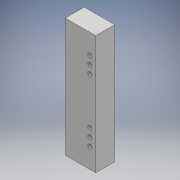
# Autodesk Inventor part: RodBase
Saved by Autodesk Inventor 2017 SP1 (Build 210196100, 196)
## iProperties
Created: 2017-10-17
Part Number: RodBase
Material: Generic
Document SubType Name: Modeling
Designer: 1452927
Density: 1 g/cm^3
Appearance: Default
Author: 1452927
Autodesk Inventor part; units mm, degrees
ref_plane "YZ Plane" through (0, 0, 0) normal (1, 0, 0) x (0, 1, 0)
ref_plane "XZ Plane" through (0, 0, 0) normal (0, 1, 0) x (-1, 0, 0)
ref_plane "XY Plane" through (0, 0, 0) normal (0, 0, 1) x (1, 0, 0)
sketch "Sketch1" plane through (0, 0, 0) normal (0, 1, 0) x (-1, 0, 0)
  line L0 (19.05, -83) -> (19.05, 83)
  line L1 (-19.05, 83) -> (-19.05, -83)
  circle A0 centre (0, 0) radius 11.5094
  line L2 (0, 0) -> (-0.4877, 3.251) construction
  line L3 (0, 0) -> (0, 44.45) construction
  line L4 (0, 0) -> (0, -44.45) construction
  circle A1 centre (0, 44.45) radius 3.5719
  circle A2 centre (0, -44.45) radius 3.5719
  line L5 (19.05, 83) -> (-19.05, 83)
  line L6 (19.05, -83) -> (-19.05, -83)
  dimension "d2" = 23.0188
  dimension "d4" = 44.45
  dimension "d5" = 44.45
  dimension "d6" = 7.1437
  dimension "d7" = 7.1437
  constraints: 14 end point, 3 centre point, 3 coincident, 2 perpendicular, 2 vertical, 1 parallel
  measures "d2" diameter of A0
  measures "d4" distance of L2.start L3.end
  measures "d5" distance of L2.start L4.end
  measures "d6" diameter of A1
  measures "d7" diameter of A2
extrude "Extrusion1" add sketch "Sketch1" along normal blind 25.4
sketch "Sketch6" plane through (0, 0, 0) normal (0, -1, 0) x (1, 0, 0)
  circle A0 centre (0, 44.45) radius 3.5719 projected
  circle A1 centre (0, 44.45) radius 3.5719
  circle A2 centre (0, -44.45) radius 3.5719 projected
  circle A3 centre (0, -44.45) radius 3.5719
  circle A4 centre (0, 0) radius 5.1594
  circle A5 centre (0, 0) radius 11.5094
  dimension "d102" = 35.7188
  constraints: 4 centre point, 4 coincident
sketch "Sketch13" plane through (0, 25.4, 0) normal (0, 1, 0) x (1, 0, 0)
  line L0 (-19.05, -83) -> (19.05, -83) construction
  line L1 (19.05, 83) -> (-19.05, 83) construction
  circle A0 centre (8.0969, -34) radius 1.8
  circle A1 centre (8.0969, -27) radius 1.8
  circle A2 centre (8.0969, -20) radius 1.8
  circle A3 centre (8.0969, 20) radius 1.8
  circle A4 centre (8.0969, 27) radius 1.8
  circle A5 centre (8.0969, 34) radius 1.8
  circle A6 centre (0, 0) radius 11.5094 projected
  line L2 (-19.05, 83) -> (-19.05, -83) projected
  line L3 (-19.05, -83) -> (-13.0969, -83)
  line L4 (-13.0969, -83) -> (-13.0969, 83)
  line L5 (-13.0969, 83) -> (-19.05, 83)
  line L6 (-19.05, 83) -> (-19.05, -83)
  line L7 (19.05, -83) -> (13.0969, -83)
  line L8 (13.0969, -83) -> (13.0969, 83)
  line L9 (13.0969, 83) -> (19.05, 83)
  line L10 (19.05, 83) -> (19.05, -83)
  line L11 (13.0969, -83) -> (3.0969, -83) construction
  line L12 (3.0969, -83) -> (3.0969, 83) construction
  line L13 (3.0969, 83) -> (13.0969, 83) construction
  line L14 (13.0969, 83) -> (13.0969, -83) construction
  line L15 (8.0969, -83) -> (8.0969, 83) construction
  dimension "d82" = 3.6
  dimension "d83" = 3.6
  dimension "d84" = 3.6
  dimension "d85" = 3.6
  dimension "d86" = 3.6
  dimension "d87" = 3.6
  dimension "d88" = 7
  dimension "d89" = 7
  dimension "d90" = 7
  dimension "d92" = 7
  dimension "d93" = 20
  dimension "d94" = 20
  dimension "d97" = 1.5875
  dimension "d99" = 1.5875
  dimension "d105" = 10
  constraints: 26 end point, 6 centre point, 6 parallel, 6 point on line, 3 horizontal, 3 perpendicular, 2 midpoint
  measures "d82" diameter of A0
  measures "d83" diameter of A1
  measures "d84" diameter of A2
  measures "d85" diameter of A3
  measures "d86" diameter of A4
  measures "d87" diameter of A5
  measures "d88" distance of A1.centre A0.centre
  measures "d89" distance of A2.centre A1.centre
  measures "d90" distance of A4.centre A3.centre
  measures "d92" distance of A5.centre A4.centre
  measures "d93" vertical distance of A6.centre A3.centre
  measures "d94" vertical distance of A2.centre A6.centre
  measures "d97" distance edge to line of A6 L4
  measures "d99" distance edge to line of A6 L8
  measures "d105" distance between parallel lines of L8 L12
sketch "Sketch14" plane through (19.05, 0, -83) normal (0, 0, -1) x (-1, 0, 0)
  line L0 (0, 0) -> (0, 25.4) projected
  line L1 (38.1, 0) -> (38.1, 25.4) projected
  line L2 (0, 25.4) -> (38.1, 25.4)
  line L3 (38.1, 25.4) -> (38.1, 16.2292)
  line L4 (38.1, 16.2292) -> (0, 16.2292)
  line L5 (0, 16.2292) -> (0, 25.4)
  point P0 (19.05, 0)
  constraints: 8 end point, 2 parallel, 1 horizontal, 1 perpendicular, 1 point on line
extrude "Extrusion15" cut sketch "Sketch14" against normal up to next
sketch "Sketch15" plane through (-19.05, 16.2292, -83) normal (0, 1, 0) x (1, 0, 0)
  line L0 (38.1, -166) -> (0, -166) projected
  line L1 (38.1, 0) -> (38.1, -166) projected
  line L2 (0, -166) -> (38.1, -166)
  line L3 (38.1, -166) -> (38.1, -134.1969)
  line L4 (38.1, -134.1969) -> (0, -134.1969)
  line L5 (0, -134.1969) -> (0, -166)
  circle A0 centre (19.05, -127.45) radius 3.5719 projected
  line L6 (0, -166) -> (0, 0) projected
  line L7 (0, 0) -> (38.1, 0)
  line L8 (38.1, 0) -> (38.1, -31.8031)
  line L9 (38.1, -31.8031) -> (0, -31.8031)
  line L10 (0, -31.8031) -> (0, 0)
  circle A1 centre (19.05, -38.55) radius 3.5719 projected
  point P0 (19.05, -83)
  dimension "d78" = 3.175
  dimension "d79" = 3.175
  constraints: 16 end point, 4 parallel, 2 horizontal, 2 perpendicular, 2 point on line
  measures "d78" distance edge to line of A0 L4
  measures "d79" distance edge to line of A1 L9
extrude "Extrusion16" cut sketch "Sketch15" against normal up to next contours L0 L5 L4 L1 | L9 L6 L7 L1
extrude "Extrusion18" cut sketch "Sketch13" against normal up to next contours A0 | A1 | A2 | A3 | A4 | A5 | L5 L4 L3 L2 | L7 L8 L9 L10
extrude "Extrusion19" add sketch "Sketch6" against normal blind 5 contours A0 | A2 | A4 | A5
body "Solid1"
